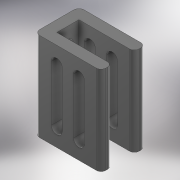
# Autodesk Inventor part: VerticalBeamMount
Saved by Autodesk Inventor 2020.3 (Build 243373000, 373)
## iProperties
Created: 2021-08-03
Part Number: VerticalBeamMount
Material: ABS Plastic
Document SubType Name: Modeling
Designer: justi
Density: 1.06 g/cm^3
Appearance: Smooth - Black
Author: justi
Autodesk Inventor part; units mm, degrees
ref_plane "YZ Plane" through (0, 0, 0) normal (1, 0, 0) x (0, 1, 0)
ref_plane "XZ Plane" through (0, 0, 0) normal (0, 1, 0) x (-1, 0, 0)
ref_plane "XY Plane" through (0, 0, 0) normal (0, 0, 1) x (1, 0, 0)
sketch "Sketch1" plane through (0, 0, 0) normal (0, 1, 0) x (-1, 0, 0)
  line L0 (20, 10) -> (-20, 10)
  line L1 (-20, 10) -> (-20, -10)
  line L2 (-20, -10) -> (20, -10)
  line L3 (20, -10) -> (20, 10)
  line L4 (20, 10) -> (-20, -10) construction
  line L5 (-20, 10) -> (20, -10) construction
  line L6 (-30, 20) -> (30, 20)
  line L7 (30, 20) -> (30, -20)
  line L8 (30, -20) -> (-30, -20)
  line L9 (-30, -20) -> (-30, 20)
  line L10 (30, 0) -> (-30, 0) construction
  line L11 (-20, 0) -> (-10, 0) construction
  line L12 (-10, 10) -> (-10, -10) construction
  line L13 (20, 10) -> (10, 10) construction
  line L14 (10, 10) -> (10, -10) construction
  point P0 (0, 0)
  dimension "d0" = 40
  dimension "d1" = 20
  dimension "d2" = 10
  dimension "d3" = 10
  dimension "d4" = 10
  constraints: 30 end point, 6 point on line, 5 midpoint, 4 parallel, 4 perpendicular, 1 horizontal, 3 other
  measures "d0" distance of L2.end L1.end
  measures "d1" distance of L1.end L0.end
  measures "d2" distance between parallel lines of L0 L6
  measures "d3" distance of L11.start L11.end
  measures "d4" distance of L0.start L13.end
extrude "Extrusion1" add sketch "Sketch1" along normal blind 80
sketch "Sketch2" plane through (-30, 0, 20) normal (0, 0, 1) x (1, 0, 0)
  line L0 (0, 0) -> (0, 80) projected
  line L1 (0, 40) -> (20, 40) construction
  line L2 (60, 0) -> (60, 80) projected
  line L3 (60, 40) -> (40, 40) construction
  line L4 (50, 0) -> (10, 0) projected
  line L5 (20, 0) -> (20, 70) construction
  line L6 (40, 0) -> (40, 80) construction
  line L7 (60, 80) -> (0, 80) projected
  line L8 (20, 65) -> (20, 15) construction
  line L9 (15.1, 65) -> (15.1, 15)
  line L10 (24.9, 15) -> (24.9, 65)
  arc A0 (24.9, 65) -> (15.1, 65) centre (20, 65) ccw
  arc A1 (15.1, 15) -> (24.9, 15) centre (20, 15) ccw
  line L11 (40, 65) -> (40, 15) construction
  line L12 (35.1, 65) -> (35.1, 15)
  line L13 (44.9, 15) -> (44.9, 65)
  arc A2 (44.9, 65) -> (35.1, 65) centre (40, 65) ccw
  arc A3 (35.1, 15) -> (44.9, 15) centre (40, 15) ccw
  point P0 (30, 0)
  dimension "d7" = 20
  dimension "d8" = 20
  dimension "d9" = 25
  dimension "d10" = 9.8
  dimension "d11" = 9.8
  constraints: 24 end point, 8 point on circle, 8 tangent, 4 centre point, 4 midpoint, 4 point on line, 2 horizontal, 2 parallel, 2 vertical, 2 other
  measures "d7" distance of L1.start L1.end
  measures "d8" distance of L3.start L3.end
  measures "d9" distance of L1.end L8.end
  measures "d10" diameter of A1
  measures "d11" diameter of A3
extrude "Extrusion2" cut sketch "Sketch2" against normal through all
sketch "Sketch3" plane through (-30, 0, -20) normal (-1, 0, 0) x (0, 0, 1)
  line L0 (20, 0) -> (20, 79.4763) construction
  line L1 (20, 64.7382) -> (20, 14.7382) construction
  line L2 (15.1, 64.7382) -> (15.1, 14.7382)
  line L3 (24.9, 14.7382) -> (24.9, 64.7382)
  arc A0 (24.9, 64.7382) -> (15.1, 64.7382) centre (20, 64.7382) ccw
  arc A1 (15.1, 14.7382) -> (24.9, 14.7382) centre (20, 14.7382) ccw
  point P0 (20, 39.7382)
  dimension "d14" = 25
  dimension "d15" = 9.8
  constraints: 10 end point, 4 point on circle, 4 tangent, 2 centre point, 2 midpoint, 1 parallel, 1 point on line, 1 vertical
  measures "d14" distance of point (20, 39.738) L1.end
  measures "d15" diameter of A1
extrude "Extrusion3" cut sketch "Sketch3" against normal blind 10
sketch "Sketch5" plane through (0, 80, 0) normal (0, 1, 0) x (1, 0, 0)
  line L0 (-20, 10) -> (20, 10) projected
  line L1 (30, -20) -> (30, 20) projected
  line L2 (20, 10) -> (30, 10)
  line L3 (30, 10) -> (30, -10)
  line L4 (30, -10) -> (20, -10)
  line L5 (20, -10) -> (20, 10)
  point P0 (0, 0)
  dimension "d18" = 20
  constraints: 8 end point, 2 parallel, 1 horizontal, 1 perpendicular, 1 point on line
  measures "d18" distance of L2.end L3.end
extrude "Extrusion4" cut sketch "Sketch5" against normal through all
fillet "Fillet1" radius 4.25 4 edges at (30, 40, 10) (30, 40, -10) (30, 40, -20) (30, 40, 20)
fillet "Fillet2" radius 4.75 2 edges at (-30, 40, 20) (-30, 40, -20)
body "Solid1"
